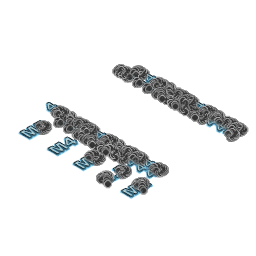
Screw-Measuring-Tool-50mm-M5_labels-only (Autodesk Fusion 360 design; units mm, degrees)
Autodesk Fusion 360 part; units mm, degrees
(part 1 of 3)
sketch "sketch 3553" plane through (0, 0, 10) normal (0, 0, 1) x (1, 0, 0)
  line L0 (16.5014, -8.6639) -> (16.5014, -9.6)
  line L1 (16.5014, -9.6) -> (15.3999, -8.6639)
  line L2 (15.3999, -8.6639) -> (16.5014, -8.6639)
  line L3 (17.91, -7.8164) -> (17.91, -8.6639)
  line L4 (17.2558, -7.8164) -> (17.91, -7.8164)
  line L5 (17.2558, -7.3771) -> (17.2558, -7.8164)
  line L6 (16.5014, -7.3771) -> (17.2558, -7.3771)
  line L7 (16.5014, -7.8164) -> (16.5014, -7.3771)
  line L8 (14.3503, -7.8164) -> (16.5014, -7.8164)
  line L9 (14.3503, -8.6639) -> (14.3503, -7.8164)
  line L10 (16.456, -10.4354) -> (14.3503, -8.6639)
  line L11 (17.2558, -10.4354) -> (16.456, -10.4354)
  line L12 (17.2558, -8.6639) -> (17.2558, -10.4354)
  line L13 (17.91, -8.6639) -> (17.2558, -8.6639)
  line L14 (16.5014, -11.9252) -> (16.5014, -12.8612)
  line L15 (16.5014, -12.8612) -> (15.3999, -11.9252)
  line L16 (15.3999, -11.9252) -> (16.5014, -11.9252)
  line L17 (17.91, -11.0777) -> (17.91, -11.9252)
  line L18 (17.2558, -11.0777) -> (17.91, -11.0777)
  line L19 (17.2558, -10.6384) -> (17.2558, -11.0777)
  line L20 (16.5014, -10.6384) -> (17.2558, -10.6384)
  line L21 (16.5014, -11.0777) -> (16.5014, -10.6384)
  line L22 (14.3503, -11.0777) -> (16.5014, -11.0777)
  line L23 (14.3503, -11.9252) -> (14.3503, -11.0777)
  line L24 (16.456, -13.6967) -> (14.3503, -11.9252)
  line L25 (17.2558, -13.6967) -> (16.456, -13.6967)
  line L26 (17.2558, -11.9252) -> (17.2558, -13.6967)
  line L27 (17.91, -11.9252) -> (17.2558, -11.9252)
  line L28 (-3.4986, -8.6639) -> (-3.4986, -9.6)
  line L29 (-3.4986, -9.6) -> (-4.6001, -8.6639)
  line L30 (-4.6001, -8.6639) -> (-3.4986, -8.6639)
  line L31 (-2.09, -7.8164) -> (-2.09, -8.6639)
  line L32 (-2.7442, -7.8164) -> (-2.09, -7.8164)
  line L33 (-2.7442, -7.3771) -> (-2.7442, -7.8164)
  line L34 (-3.4986, -7.3771) -> (-2.7442, -7.3771)
  line L35 (-3.4986, -7.8164) -> (-3.4986, -7.3771)
  line L36 (-5.6497, -7.8164) -> (-3.4986, -7.8164)
  line L37 (-5.6497, -8.6639) -> (-5.6497, -7.8164)
  line L38 (-3.544, -10.4354) -> (-5.6497, -8.6639)
  line L39 (-2.7442, -10.4354) -> (-3.544, -10.4354)
  line L40 (-2.7442, -8.6639) -> (-2.7442, -10.4354)
  line L41 (-2.09, -8.6639) -> (-2.7442, -8.6639)
  spline S0 degree 2 poles (-13.0958, -12.5579) (-13.3202, -12.2833) (-13.6497, -12.1281) knots 0 0 0 1 1 1
  spline S1 degree 2 poles (-12.7114, -13.329) (-12.8714, -12.8324) (-13.0958, -12.5579) knots 0 0 0 1 1 1
  line L42 (-11.914, -13.329) -> (-12.7114, -13.329)
  spline S2 degree 2 poles (-12.1289, -12.7692) (-12.0167, -12.9924) (-11.914, -13.329) knots 0 0 0 1 1 1
  spline S3 degree 2 poles (-12.4225, -12.3072) (-12.2411, -12.5459) (-12.1289, -12.7692) knots 0 0 0 1 1 1
  line L43 (-10.09, -12.3072) -> (-12.4225, -12.3072)
  line L44 (-10.09, -11.3236) -> (-10.09, -12.3072)
  line L45 (-13.6497, -11.3236) -> (-10.09, -11.3236)
  line L46 (-13.6497, -12.1281) -> (-13.6497, -11.3236)
  line L47 (-14.8826, -8.8955) -> (-14.8826, -7.3771)
  spline S4 degree 2 poles (-15.0951, -8.6627) (-15.0139, -8.7618) (-14.8826, -8.8955) knots 0 0 0 1 1 1
  spline S5 degree 2 poles (-15.3792, -8.27) (-15.1763, -8.5637) (-15.0951, -8.6627) knots 0 0 0 1 1 1
  spline S6 degree 2 poles (-16.0191, -7.5884) (-15.7278, -7.7758) (-15.3792, -8.27) knots 0 0 0 1 1 1
  spline S7 degree 2 poles (-16.6302, -7.401) (-16.3103, -7.401) (-16.0191, -7.5884) knots 0 0 0 1 1 1
  spline S8 degree 2 poles (-17.1734, -7.5645) (-16.9311, -7.401) (-16.6302, -7.401) knots 0 0 0 1 1 1
  spline S9 degree 2 poles (-17.5327, -8.0134) (-17.4157, -7.7281) (-17.1734, -7.5645) knots 0 0 0 1 1 1
  spline S10 degree 2 poles (-17.6497, -8.812) (-17.6497, -8.2987) (-17.5327, -8.0134) knots 0 0 0 1 1 1
  spline S11 degree 2 poles (-17.5267, -9.5819) (-17.6497, -9.3038) (-17.6497, -8.812) knots 0 0 0 1 1 1
  spline S12 degree 2 poles (-17.1734, -10.0129) (-17.4038, -9.8601) (-17.5267, -9.5819) knots 0 0 0 1 1 1
  spline S13 degree 2 poles (-16.5324, -10.2229) (-16.943, -10.1656) (-17.1734, -10.0129) knots 0 0 0 1 1 1
  line L48 (-16.4536, -9.2489) -> (-16.5324, -10.2229)
  spline S14 degree 2 poles (-16.8666, -9.0901) (-16.7496, -9.2083) (-16.4536, -9.2489) knots 0 0 0 1 1 1
  spline S15 degree 2 poles (-16.9836, -8.7857) (-16.9836, -8.9719) (-16.8666, -9.0901) knots 0 0 0 1 1 1
  spline S16 degree 2 poles (-16.8702, -8.4885) (-16.9836, -8.6066) (-16.9836, -8.7857) knots 0 0 0 1 1 1
  spline S17 degree 2 poles (-16.5968, -8.3703) (-16.7568, -8.3703) (-16.8702, -8.4885) knots 0 0 0 1 1 1
  spline S18 degree 2 poles (-16.2841, -8.4897) (-16.4488, -8.3703) (-16.5968, -8.3703) knots 0 0 0 1 1 1
  spline S19 degree 2 poles (-15.8018, -9.0364) (-16.1193, -8.609) (-16.2841, -8.4897) knots 0 0 0 1 1 1
  spline S20 degree 2 poles (-14.9029, -9.9902) (-15.2837, -9.7359) (-15.8018, -9.0364) knots 0 0 0 1 1 1
  spline S21 degree 2 poles (-14.09, -10.2946) (-14.5221, -10.2444) (-14.9029, -9.9902) knots 0 0 0 1 1 1
  line L49 (-14.09, -7.3771) -> (-14.09, -10.2946)
  line L50 (-14.8826, -7.3771) -> (-14.09, -7.3771)
  spline S22 degree 2 poles (-20.6589, -9.2154) (-20.8356, -9.2154) (-20.9466, -9.1044) knots -1 -1 -1 0 0 0
  spline S23 degree 2 poles (-20.9466, -9.1044) (-21.0576, -8.9934) (-21.0576, -8.8167) knots -1 -1 -1 0 0 0
  spline S24 degree 2 poles (-21.0576, -8.8167) (-21.0576, -8.6425) (-20.9442, -8.5302) knots -1 -1 -1 0 0 0
  spline S25 degree 2 poles (-20.9442, -8.5302) (-20.8308, -8.418) (-20.6493, -8.418) knots -1 -1 -1 0 0 0
  spline S26 degree 2 poles (-20.6493, -8.418) (-20.4751, -8.418) (-20.3652, -8.5255) knots -1 -1 -1 0 0 0
  spline S27 degree 2 poles (-20.3652, -8.5255) (-20.2554, -8.6329) (-20.2554, -8.8) knots -1 -1 -1 0 0 0
  spline S28 degree 2 poles (-20.2554, -8.8) (-20.2554, -8.9886) (-20.3664, -9.102) knots -1 -1 -1 0 0 0
  spline S29 degree 2 poles (-20.3664, -9.102) (-20.4774, -9.2154) (-20.6589, -9.2154) knots -1 -1 -1 0 0 0
  spline S30 degree 2 poles (-19.1524, -9.268) (-19.3959, -9.268) (-19.5392, -9.1331) knots -1 -1 -1 0 0 0
  spline S31 degree 2 poles (-19.5392, -9.1331) (-19.6824, -8.9982) (-19.6824, -8.8167) knots -1 -1 -1 0 0 0
  spline S32 degree 2 poles (-19.6824, -8.8167) (-19.6824, -8.6329) (-19.5344, -8.4932) knots -1 -1 -1 0 0 0
  spline S33 degree 2 poles (-19.5344, -8.4932) (-19.3864, -8.3536) (-19.1548, -8.3536) knots -1 -1 -1 0 0 0
  spline S34 degree 2 poles (-19.1548, -8.3536) (-18.9256, -8.3536) (-18.7764, -8.492) knots -1 -1 -1 0 0 0
  spline S35 degree 2 poles (-18.7764, -8.492) (-18.6272, -8.6305) (-18.6272, -8.8048) knots -1 -1 -1 0 0 0
  spline S36 degree 2 poles (-18.6272, -8.8048) (-18.6272, -8.9862) (-18.774, -9.1271) knots -1 -1 -1 0 0 0
  spline S37 degree 2 poles (-18.774, -9.1271) (-18.9208, -9.268) (-19.1524, -9.268) knots -1 -1 -1 0 0 0
  spline S38 degree 2 poles (-19.119, -10.2373) (-19.427, -10.2373) (-19.6406, -10.094) knots 0 0 0 1 1 1
  spline S39 degree 2 poles (-18.5484, -10.0845) (-18.8038, -10.2373) (-19.119, -10.2373) knots 0 0 0 1 1 1
  spline S40 degree 2 poles (-18.1616, -9.638) (-18.2929, -9.9317) (-18.5484, -10.0845) knots 0 0 0 1 1 1
  spline S41 degree 2 poles (-18.0303, -8.7881) (-18.0303, -9.3444) (-18.1616, -9.638) knots 0 0 0 1 1 1
  spline S42 degree 2 poles (-18.0888, -8.2306) (-18.0303, -8.492) (-18.0303, -8.7881) knots 0 0 0 1 1 1
  spline S43 degree 2 poles (-18.2714, -7.7937) (-18.1473, -7.9692) (-18.0888, -8.2306) knots 0 0 0 1 1 1
  spline S44 degree 2 poles (-18.6236, -7.4977) (-18.3956, -7.6182) (-18.2714, -7.7937) knots 0 0 0 1 1 1
  spline S45 degree 2 poles (-19.1142, -7.3771) (-18.8516, -7.3771) (-18.6236, -7.4977) knots 0 0 0 1 1 1
  spline S46 degree 2 poles (-19.6108, -7.5168) (-19.3864, -7.3771) (-19.1142, -7.3771) knots 0 0 0 1 1 1
  spline S47 degree 2 poles (-19.9713, -7.9405) (-19.8352, -7.6564) (-19.6108, -7.5168) knots 0 0 0 1 1 1
  spline S48 degree 2 poles (-20.2674, -7.6254) (-20.1146, -7.7257) (-19.9713, -7.9405) knots 0 0 0 1 1 1
  spline S49 degree 2 poles (-20.709, -7.4917) (-20.4727, -7.4917) (-20.2674, -7.6254) knots 0 0 0 1 1 1
  spline S50 degree 2 poles (-21.3823, -7.8271) (-21.1149, -7.4917) (-20.709, -7.4917) knots 0 0 0 1 1 1
  spline S51 degree 2 poles (-21.6497, -8.8645) (-21.6497, -8.1626) (-21.3823, -7.8271) knots 0 0 0 1 1 1
  spline S52 degree 2 poles (-21.4348, -9.7168) (-21.6497, -9.3945) (-21.6497, -8.8645) knots 0 0 0 1 1 1
  spline S53 degree 2 poles (-20.7162, -10.1298) (-21.1555, -10.1298) (-21.4348, -9.7168) knots 0 0 0 1 1 1
  spline S54 degree 2 poles (-20.2435, -9.9866) (-20.4488, -10.1298) (-20.7162, -10.1298) knots 0 0 0 1 1 1
  spline S55 degree 2 poles (-19.9713, -9.6523) (-20.0931, -9.8815) (-20.2435, -9.9866) knots 0 0 0 1 1 1
  spline S56 degree 2 poles (-19.6406, -10.094) (-19.8543, -9.9508) (-19.9713, -9.6523) knots 0 0 0 1 1 1
  line L51 (1.1174, -12.1711) -> (1.1174, -10.6527)
  spline S57 degree 2 poles (0.9049, -11.9383) (0.9861, -12.0374) (1.1174, -12.1711) knots 0 0 0 1 1 1
  spline S58 degree 2 poles (0.6208, -11.5456) (0.8237, -11.8392) (0.9049, -11.9383) knots 0 0 0 1 1 1
  spline S59 degree 2 poles (-0.0191, -10.864) (0.2722, -11.0514) (0.6208, -11.5456) knots 0 0 0 1 1 1
  spline S60 degree 2 poles (-0.6302, -10.6766) (-0.3103, -10.6766) (-0.0191, -10.864) knots 0 0 0 1 1 1
  spline S61 degree 2 poles (-1.1734, -10.8401) (-0.9311, -10.6766) (-0.6302, -10.6766) knots 0 0 0 1 1 1
  spline S62 degree 2 poles (-1.5327, -11.2889) (-1.4157, -11.0036) (-1.1734, -10.8401) knots 0 0 0 1 1 1
  spline S63 degree 2 poles (-1.6497, -12.0875) (-1.6497, -11.5742) (-1.5327, -11.2889) knots 0 0 0 1 1 1
  spline S64 degree 2 poles (-1.5267, -12.8575) (-1.6497, -12.5794) (-1.6497, -12.0875) knots 0 0 0 1 1 1
  spline S65 degree 2 poles (-1.1734, -13.2884) (-1.4038, -13.1356) (-1.5267, -12.8575) knots 0 0 0 1 1 1
  spline S66 degree 2 poles (-0.5324, -13.4985) (-0.943, -13.4412) (-1.1734, -13.2884) knots 0 0 0 1 1 1
  line L52 (-0.4536, -12.5244) -> (-0.5324, -13.4985)
  spline S67 degree 2 poles (-0.8666, -12.3657) (-0.7496, -12.4839) (-0.4536, -12.5244) knots 0 0 0 1 1 1
  spline S68 degree 2 poles (-0.9836, -12.0613) (-0.9836, -12.2475) (-0.8666, -12.3657) knots 0 0 0 1 1 1
  spline S69 degree 2 poles (-0.8702, -11.764) (-0.9836, -11.8822) (-0.9836, -12.0613) knots 0 0 0 1 1 1
  spline S70 degree 2 poles (-0.5968, -11.6459) (-0.7568, -11.6459) (-0.8702, -11.764) knots 0 0 0 1 1 1
  spline S71 degree 2 poles (-0.2841, -11.7652) (-0.4488, -11.6459) (-0.5968, -11.6459) knots 0 0 0 1 1 1
  spline S72 degree 2 poles (0.1982, -12.312) (-0.1193, -11.8846) (-0.2841, -11.7652) knots 0 0 0 1 1 1
  spline S73 degree 2 poles (1.0971, -13.2657) (0.7163, -13.0115) (0.1982, -12.312) knots 0 0 0 1 1 1
  spline S74 degree 2 poles (1.91, -13.5701) (1.4779, -13.52) (1.0971, -13.2657) knots 0 0 0 1 1 1
  line L53 (1.91, -10.6527) -> (1.91, -13.5701)
  line L54 (1.1174, -10.6527) -> (1.91, -10.6527)
  spline S75 degree 2 poles (6.9543, -12.1592) (6.9543, -12.3311) (7.0582, -12.4385) knots 0 0 0 1 1 1
  spline S76 degree 2 poles (7.0498, -11.8965) (6.9543, -11.992) (6.9543, -12.1592) knots 0 0 0 1 1 1
  spline S77 degree 2 poles (7.3053, -11.801) (7.1453, -11.801) (7.0498, -11.8965) knots 0 0 0 1 1 1
  spline S78 degree 2 poles (7.5942, -11.9288) (7.4724, -11.801) (7.3053, -11.801) knots 0 0 0 1 1 1
  spline S79 degree 2 poles (7.7159, -12.2475) (7.7159, -12.0565) (7.5942, -11.9288) knots 0 0 0 1 1 1
  spline S80 degree 2 poles (7.704, -12.374) (7.7159, -12.2929) (7.7159, -12.2475) knots 0 0 0 1 1 1
  line L55 (8.3987, -12.4242) -> (7.704, -12.374)
  spline S81 degree 2 poles (8.3414, -12.109) (8.3414, -12.2236) (8.3987, -12.4242) knots 0 0 0 1 1 1
  spline S82 degree 2 poles (8.4751, -11.7688) (8.3414, -11.8942) (8.3414, -12.109) knots 0 0 0 1 1 1
  spline S83 degree 2 poles (8.8524, -11.6435) (8.6088, -11.6435) (8.4751, -11.7688) knots 0 0 0 1 1 1
  spline S84 degree 2 poles (9.2344, -11.7736) (9.0911, -11.6435) (8.8524, -11.6435) knots 0 0 0 1 1 1
  spline S85 degree 2 poles (9.3776, -12.0995) (9.3776, -11.9037) (9.2344, -11.7736) knots 0 0 0 1 1 1
  spline S86 degree 2 poles (9.2642, -12.4063) (9.3776, -12.2857) (9.3776, -12.0995) knots 0 0 0 1 1 1
  spline S87 degree 2 poles (8.8571, -12.5841) (9.1508, -12.5268) (9.2642, -12.4063) knots 0 0 0 1 1 1
  line L56 (8.9861, -13.5558) -> (8.8571, -12.5841)
  spline S88 degree 2 poles (9.5292, -13.2825) (9.3131, -13.4603) (8.9861, -13.5558) knots 0 0 0 1 1 1
  spline S89 degree 2 poles (9.8575, -12.8288) (9.7453, -13.1046) (9.5292, -13.2825) knots 0 0 0 1 1 1
  spline S90 degree 2 poles (9.9697, -12.0756) (9.9697, -12.5531) (9.8575, -12.8288) knots 0 0 0 1 1 1
  spline S91 degree 2 poles (9.8181, -11.2854) (9.9697, -11.5862) (9.9697, -12.0756) knots 0 0 0 1 1 1
  spline S92 degree 2 poles (9.386, -10.8246) (9.6665, -10.9845) (9.8181, -11.2854) knots 0 0 0 1 1 1
  spline S93 degree 2 poles (8.7998, -10.6646) (9.1054, -10.6646) (9.386, -10.8246) knots 0 0 0 1 1 1
  spline S94 degree 2 poles (8.3808, -10.7613) (8.5563, -10.6646) (8.7998, -10.6646) knots 0 0 0 1 1 1
  spline S95 degree 2 poles (8.0979, -11.0323) (8.2054, -10.858) (8.3808, -10.7613) knots 0 0 0 1 1 1
  spline S96 degree 2 poles (7.9809, -11.3427) (8.0311, -11.1397) (8.0979, -11.0323) knots 0 0 0 1 1 1
  spline S97 degree 2 poles (7.6586, -10.9678) (7.8425, -11.092) (7.9809, -11.3427) knots 0 0 0 1 1 1
  spline S98 degree 2 poles (7.248, -10.8437) (7.4748, -10.8437) (7.6586, -10.9678) knots 0 0 0 1 1 1
  spline S99 degree 2 poles (6.6058, -11.1493) (6.8612, -10.8437) (7.248, -10.8437) knots 0 0 0 1 1 1
  spline S100 degree 2 poles (6.3503, -12.1401) (6.3503, -11.4549) (6.6058, -11.1493) knots 0 0 0 1 1 1
  spline S101 degree 2 poles (6.5843, -13.0628) (6.3503, -12.7369) (6.3503, -12.1401) knots 0 0 0 1 1 1
  spline S102 degree 2 poles (7.2575, -13.5033) (6.8183, -13.3887) (6.5843, -13.0628) knots 0 0 0 1 1 1
  line L57 (7.4223, -12.5841) -> (7.2575, -13.5033)
  spline S103 degree 2 poles (7.0582, -12.4385) (7.162, -12.5459) (7.4223, -12.5841) knots 0 0 0 1 1 1
  spline S104 degree 2 poles (20.8476, -9.268) (20.6041, -9.268) (20.4608, -9.1331) knots -1 -1 -1 0 0 0
  spline S105 degree 2 poles (20.4608, -9.1331) (20.3176, -8.9982) (20.3176, -8.8167) knots -1 -1 -1 0 0 0
  spline S106 degree 2 poles (20.3176, -8.8167) (20.3176, -8.6329) (20.4656, -8.4932) knots -1 -1 -1 0 0 0
  spline S107 degree 2 poles (20.4656, -8.4932) (20.6136, -8.3536) (20.8452, -8.3536) knots -1 -1 -1 0 0 0
  spline S108 degree 2 poles (20.8452, -8.3536) (21.0744, -8.3536) (21.2236, -8.492) knots -1 -1 -1 0 0 0
  spline S109 degree 2 poles (21.2236, -8.492) (21.3728, -8.6305) (21.3728, -8.8048) knots -1 -1 -1 0 0 0
  spline S110 degree 2 poles (21.3728, -8.8048) (21.3728, -8.9862) (21.226, -9.1271) knots -1 -1 -1 0 0 0
  spline S111 degree 2 poles (21.226, -9.1271) (21.0792, -9.268) (20.8476, -9.268) knots -1 -1 -1 0 0 0
  spline S112 degree 2 poles (19.3411, -9.2154) (19.1644, -9.2154) (19.0534, -9.1044) knots -1 -1 -1 0 0 0
  spline S113 degree 2 poles (19.0534, -9.1044) (18.9424, -8.9934) (18.9424, -8.8167) knots -1 -1 -1 0 0 0
  spline S114 degree 2 poles (18.9424, -8.8167) (18.9424, -8.6425) (19.0558, -8.5302) knots -1 -1 -1 0 0 0
  spline S115 degree 2 poles (19.0558, -8.5302) (19.1692, -8.418) (19.3507, -8.418) knots -1 -1 -1 0 0 0
  spline S116 degree 2 poles (19.3507, -8.418) (19.5249, -8.418) (19.6348, -8.5255) knots -1 -1 -1 0 0 0
  spline S117 degree 2 poles (19.6348, -8.5255) (19.7446, -8.6329) (19.7446, -8.8) knots -1 -1 -1 0 0 0
  spline S118 degree 2 poles (19.7446, -8.8) (19.7446, -8.9886) (19.6336, -9.102) knots -1 -1 -1 0 0 0
  spline S119 degree 2 poles (19.6336, -9.102) (19.5226, -9.2154) (19.3411, -9.2154) knots -1 -1 -1 0 0 0
  spline S120 degree 2 poles (20.881, -10.2373) (20.573, -10.2373) (20.3594, -10.094) knots 0 0 0 1 1 1
  spline S121 degree 2 poles (21.4516, -10.0845) (21.1962, -10.2373) (20.881, -10.2373) knots 0 0 0 1 1 1
  spline S122 degree 2 poles (21.8384, -9.638) (21.7071, -9.9317) (21.4516, -10.0845) knots 0 0 0 1 1 1
  spline S123 degree 2 poles (21.9697, -8.7881) (21.9697, -9.3444) (21.8384, -9.638) knots 0 0 0 1 1 1
  spline S124 degree 2 poles (21.9112, -8.2306) (21.9697, -8.492) (21.9697, -8.7881) knots 0 0 0 1 1 1
  spline S125 degree 2 poles (21.7286, -7.7937) (21.8527, -7.9692) (21.9112, -8.2306) knots 0 0 0 1 1 1
  spline S126 degree 2 poles (21.3764, -7.4977) (21.6044, -7.6182) (21.7286, -7.7937) knots 0 0 0 1 1 1
  spline S127 degree 2 poles (20.8858, -7.3771) (21.1484, -7.3771) (21.3764, -7.4977) knots 0 0 0 1 1 1
  spline S128 degree 2 poles (20.3892, -7.5168) (20.6136, -7.3771) (20.8858, -7.3771) knots 0 0 0 1 1 1
  spline S129 degree 2 poles (20.0287, -7.9405) (20.1648, -7.6564) (20.3892, -7.5168) knots 0 0 0 1 1 1
  spline S130 degree 2 poles (19.7326, -7.6254) (19.8854, -7.7257) (20.0287, -7.9405) knots 0 0 0 1 1 1
  spline S131 degree 2 poles (19.291, -7.4917) (19.5273, -7.4917) (19.7326, -7.6254) knots 0 0 0 1 1 1
  spline S132 degree 2 poles (18.6177, -7.8271) (18.8851, -7.4917) (19.291, -7.4917) knots 0 0 0 1 1 1
  spline S133 degree 2 poles (18.3503, -8.8645) (18.3503, -8.1626) (18.6177, -7.8271) knots 0 0 0 1 1 1
  spline S134 degree 2 poles (18.5652, -9.7168) (18.3503, -9.3945) (18.3503, -8.8645) knots 0 0 0 1 1 1
  spline S135 degree 2 poles (19.2838, -10.1298) (18.8445, -10.1298) (18.5652, -9.7168) knots 0 0 0 1 1 1
  spline S136 degree 2 poles (19.7565, -9.9866) (19.5512, -10.1298) (19.2838, -10.1298) knots 0 0 0 1 1 1
  spline S137 degree 2 poles (20.0287, -9.6523) (19.9069, -9.8815) (19.7565, -9.9866) knots 0 0 0 1 1 1
  spline S138 degree 2 poles (20.3594, -10.094) (20.1457, -9.9508) (20.0287, -9.6523) knots 0 0 0 1 1 1
  line L58 (-6.8826, -12.1711) -> (-6.8826, -10.6527)
  spline S139 degree 2 poles (-7.0951, -11.9383) (-7.0139, -12.0374) (-6.8826, -12.1711) knots 0 0 0 1 1 1
  spline S140 degree 2 poles (-7.3792, -11.5456) (-7.1763, -11.8392) (-7.0951, -11.9383) knots 0 0 0 1 1 1
  spline S141 degree 2 poles (-8.0191, -10.864) (-7.7278, -11.0514) (-7.3792, -11.5456) knots 0 0 0 1 1 1
  spline S142 degree 2 poles (-8.6302, -10.6766) (-8.3103, -10.6766) (-8.0191, -10.864) knots 0 0 0 1 1 1
  spline S143 degree 2 poles (-9.1734, -10.8401) (-8.9311, -10.6766) (-8.6302, -10.6766) knots 0 0 0 1 1 1
  spline S144 degree 2 poles (-9.5327, -11.2889) (-9.4157, -11.0036) (-9.1734, -10.8401) knots 0 0 0 1 1 1
  spline S145 degree 2 poles (-9.6497, -12.0875) (-9.6497, -11.5742) (-9.5327, -11.2889) knots 0 0 0 1 1 1
  spline S146 degree 2 poles (-9.5267, -12.8575) (-9.6497, -12.5794) (-9.6497, -12.0875) knots 0 0 0 1 1 1
  spline S147 degree 2 poles (-9.1734, -13.2884) (-9.4038, -13.1356) (-9.5267, -12.8575) knots 0 0 0 1 1 1
  spline S148 degree 2 poles (-8.5324, -13.4985) (-8.943, -13.4412) (-9.1734, -13.2884) knots 0 0 0 1 1 1
  line L59 (-8.4536, -12.5244) -> (-8.5324, -13.4985)
  spline S149 degree 2 poles (-8.8666, -12.3657) (-8.7496, -12.4839) (-8.4536, -12.5244) knots 0 0 0 1 1 1
  spline S150 degree 2 poles (-8.9836, -12.0613) (-8.9836, -12.2475) (-8.8666, -12.3657) knots 0 0 0 1 1 1
  spline S151 degree 2 poles (-8.8702, -11.764) (-8.9836, -11.8822) (-8.9836, -12.0613) knots 0 0 0 1 1 1
  spline S152 degree 2 poles (-8.5968, -11.6459) (-8.7568, -11.6459) (-8.8702, -11.764) knots 0 0 0 1 1 1
  spline S153 degree 2 poles (-8.2841, -11.7652) (-8.4488, -11.6459) (-8.5968, -11.6459) knots 0 0 0 1 1 1
  spline S154 degree 2 poles (-7.8018, -12.312) (-8.1193, -11.8846) (-8.2841, -11.7652) knots 0 0 0 1 1 1
  spline S155 degree 2 poles (-6.9029, -13.2657) (-7.2837, -13.0115) (-7.8018, -12.312) knots 0 0 0 1 1 1
  spline S156 degree 2 poles (-6.09, -13.5701) (-6.5221, -13.52) (-6.9029, -13.2657) knots 0 0 0 1 1 1
  line L60 (-6.09, -10.6527) -> (-6.09, -13.5701)
  line L61 (-6.8826, -10.6527) -> (-6.09, -10.6527)
  line L62 (5.1174, -8.8955) -> (5.1174, -7.3771)
  spline S157 degree 2 poles (4.9049, -8.6627) (4.9861, -8.7618) (5.1174, -8.8955) knots 0 0 0 1 1 1
  spline S158 degree 2 poles (4.6208, -8.27) (4.8237, -8.5637) (4.9049, -8.6627) knots 0 0 0 1 1 1
  spline S159 degree 2 poles (3.9809, -7.5884) (4.2722, -7.7758) (4.6208, -8.27) knots 0 0 0 1 1 1
  spline S160 degree 2 poles (3.3698, -7.401) (3.6897, -7.401) (3.9809, -7.5884) knots 0 0 0 1 1 1
  spline S161 degree 2 poles (2.8266, -7.5645) (3.0689, -7.401) (3.3698, -7.401) knots 0 0 0 1 1 1
  spline S162 degree 2 poles (2.4673, -8.0134) (2.5843, -7.7281) (2.8266, -7.5645) knots 0 0 0 1 1 1
  spline S163 degree 2 poles (2.3503, -8.812) (2.3503, -8.2987) (2.4673, -8.0134) knots 0 0 0 1 1 1
  spline S164 degree 2 poles (2.4733, -9.5819) (2.3503, -9.3038) (2.3503, -8.812) knots 0 0 0 1 1 1
  spline S165 degree 2 poles (2.8266, -10.0129) (2.5962, -9.8601) (2.4733, -9.5819) knots 0 0 0 1 1 1
  spline S166 degree 2 poles (3.4676, -10.2229) (3.057, -10.1656) (2.8266, -10.0129) knots 0 0 0 1 1 1
  line L63 (3.5464, -9.2489) -> (3.4676, -10.2229)
  spline S167 degree 2 poles (3.1334, -9.0901) (3.2504, -9.2083) (3.5464, -9.2489) knots 0 0 0 1 1 1
  spline S168 degree 2 poles (3.0164, -8.7857) (3.0164, -8.9719) (3.1334, -9.0901) knots 0 0 0 1 1 1
  spline S169 degree 2 poles (3.1298, -8.4885) (3.0164, -8.6066) (3.0164, -8.7857) knots 0 0 0 1 1 1
  spline S170 degree 2 poles (3.4032, -8.3703) (3.2432, -8.3703) (3.1298, -8.4885) knots 0 0 0 1 1 1
  spline S171 degree 2 poles (3.7159, -8.4897) (3.5512, -8.3703) (3.4032, -8.3703) knots 0 0 0 1 1 1
  spline S172 degree 2 poles (4.1982, -9.0364) (3.8807, -8.609) (3.7159, -8.4897) knots 0 0 0 1 1 1
  spline S173 degree 2 poles (5.0971, -9.9902) (4.7163, -9.7359) (4.1982, -9.0364) knots 0 0 0 1 1 1
  spline S174 degree 2 poles (5.91, -10.2946) (5.4779, -10.2444) (5.0971, -9.9902) knots 0 0 0 1 1 1
  line L64 (5.91, -7.3771) -> (5.91, -10.2946)
  line L65 (5.1174, -7.3771) -> (5.91, -7.3771)
  spline S175 degree 2 poles (-15.0958, 17.7183) (-15.3202, 17.9928) (-15.6497, 18.148) knots 0 0 0 1 1 1
  spline S176 degree 2 poles (-14.7114, 16.9471) (-14.8714, 17.4437) (-15.0958, 17.7183) knots 0 0 0 1 1 1
  line L66 (-13.914, 16.9471) -> (-14.7114, 16.9471)
  spline S177 degree 2 poles (-14.1289, 17.507) (-14.0167, 17.2837) (-13.914, 16.9471) knots 0 0 0 1 1 1
  spline S178 degree 2 poles (-14.4225, 17.9689) (-14.2411, 17.7302) (-14.1289, 17.507) knots 0 0 0 1 1 1
  line L67 (-12.09, 17.9689) -> (-14.4225, 17.9689)
  line L68 (-12.09, 18.9526) -> (-12.09, 17.9689)
  line L69 (-15.6497, 18.9526) -> (-12.09, 18.9526)
  line L70 (-15.6497, 18.148) -> (-15.6497, 18.9526)
  line L71 (-13.4986, 21.6814) -> (-13.4986, 20.7454)
  line L72 (-13.4986, 20.7454) -> (-14.6001, 21.6814)
  line L73 (-14.6001, 21.6814) -> (-13.4986, 21.6814)
  line L74 (-12.09, 22.529) -> (-12.09, 21.6814)
  line L75 (-12.7442, 22.529) -> (-12.09, 22.529)
  line L76 (-12.7442, 22.9683) -> (-12.7442, 22.529)
  line L77 (-13.4986, 22.9683) -> (-12.7442, 22.9683)
  line L78 (-13.4986, 22.529) -> (-13.4986, 22.9683)
  line L79 (-15.6497, 22.529) -> (-13.4986, 22.529)
  line L80 (-15.6497, 21.6814) -> (-15.6497, 22.529)
  line L81 (-13.544, 19.9099) -> (-15.6497, 21.6814)
  line L82 (-12.7442, 19.9099) -> (-13.544, 19.9099)
  line L83 (-12.7442, 21.6814) -> (-12.7442, 19.9099)
  line L84 (-12.09, 21.6814) -> (-12.7442, 21.6814)
  spline S179 degree 2 poles (-19.0958, 17.7183) (-19.3202, 17.9928) (-19.6497, 18.148) knots 0 0 0 1 1 1
  spline S180 degree 2 poles (-18.7114, 16.9471) (-18.8714, 17.4437) (-19.0958, 17.7183) knots 0 0 0 1 1 1
  line L85 (-17.914, 16.9471) -> (-18.7114, 16.9471)
  spline S181 degree 2 poles (-18.1289, 17.507) (-18.0167, 17.2837) (-17.914, 16.9471) knots 0 0 0 1 1 1
  spline S182 degree 2 poles (-18.4225, 17.9689) (-18.2411, 17.7302) (-18.1289, 17.507) knots 0 0 0 1 1 1
  line L86 (-16.09, 17.9689) -> (-18.4225, 17.9689)
  line L87 (-16.09, 18.9526) -> (-16.09, 17.9689)
  line L88 (-19.6497, 18.9526) -> (-16.09, 18.9526)
  line L89 (-19.6497, 18.148) -> (-19.6497, 18.9526)
  spline S183 degree 2 poles (-21.2431, 17.9665) (-21.5225, 17.9665) (-21.6729, 18.1038) knots -1 -1 -1 0 0 0
  spline S184 degree 2 poles (-21.6729, 18.1038) (-21.8233, 18.2411) (-21.8233, 18.444) knots -1 -1 -1 0 0 0
  spline S185 degree 2 poles (-21.8233, 18.444) (-21.8233, 18.6422) (-21.6681, 18.7759) knots -1 -1 -1 0 0 0
  spline S186 degree 2 poles (-21.6681, 18.7759) (-21.5129, 18.9096) (-21.2169, 18.9096) knots -1 -1 -1 0 0 0
  spline S187 degree 2 poles (-21.2169, 18.9096) (-20.928, 18.9096) (-20.7824, 18.7807) knots -1 -1 -1 0 0 0
  spline S188 degree 2 poles (-20.7824, 18.7807) (-20.6367, 18.6517) (-20.6367, 18.4607) knots -1 -1 -1 0 0 0
  spline S189 degree 2 poles (-20.6367, 18.4607) (-20.6367, 18.253) (-20.7979, 18.1098) knots -1 -1 -1 0 0 0
  spline S190 degree 2 poles (-20.7979, 18.1098) (-20.959, 17.9665) (-21.2431, 17.9665) knots -1 -1 -1 0 0 0
  spline S191 degree 2 poles (-23.553, 19.1113) (-23.4563, 19.3537) (-23.2701, 19.5136) knots 0 0 0 1 1 1
  spline S192 degree 2 poles (-23.6497, 18.4512) (-23.6497, 18.869) (-23.553, 19.1113) knots 0 0 0 1 1 1
  spline S193 degree 2 poles (-23.2092, 17.3458) (-23.6497, 17.7445) (-23.6497, 18.4512) knots 0 0 0 1 1 1
  spline S194 degree 2 poles (-21.8209, 16.9471) (-22.7687, 16.9471) (-23.2092, 17.3458) knots 0 0 0 1 1 1
  spline S195 degree 2 poles (-20.7812, 17.1369) (-21.1739, 16.9471) (-21.8209, 16.9471) knots 0 0 0 1 1 1
  spline S196 degree 2 poles (-20.2094, 17.6442) (-20.3884, 17.3267) (-20.7812, 17.1369) knots 0 0 0 1 1 1
  spline S197 degree 2 poles (-20.0303, 18.487) (-20.0303, 17.9618) (-20.2094, 17.6442) knots 0 0 0 1 1 1
  spline S198 degree 2 poles (-20.1771, 19.214) (-20.0303, 18.9239) (-20.0303, 18.487) knots 0 0 0 1 1 1
  spline S199 degree 2 poles (-20.6105, 19.6676) (-20.324, 19.5041) (-20.1771, 19.214) knots 0 0 0 1 1 1
  spline S200 degree 2 poles (-21.2431, 19.8311) (-20.897, 19.8311) (-20.6105, 19.6676) knots 0 0 0 1 1 1
  spline S201 degree 2 poles (-22.0907, 19.5076) (-21.7564, 19.8311) (-21.2431, 19.8311) knots 0 0 0 1 1 1
  spline S202 degree 2 poles (-22.4249, 18.7162) (-22.4249, 19.1841) (-22.0907, 19.5076) knots 0 0 0 1 1 1
  spline S203 degree 2 poles (-22.3402, 18.2912) (-22.4249, 18.4751) (-22.4249, 18.7162) knots 0 0 0 1 1 1
  spline S204 degree 2 poles (-22.0787, 17.9331) (-22.2554, 18.1074) (-22.3402, 18.2912) knots 0 0 0 1 1 1
  spline S205 degree 2 poles (-22.8141, 18.074) (-22.6422, 17.9785) (-22.0787, 17.9331) knots 0 0 0 1 1 1
  spline S206 degree 2 poles (-23.0528, 18.4416) (-23.0528, 18.2053) (-22.8141, 18.074) knots 0 0 0 1 1 1
  spline S207 degree 2 poles (-22.9693, 18.6625) (-23.0528, 18.573) (-23.0528, 18.4416) knots 0 0 0 1 1 1
  spline S208 degree 2 poles (-22.6828, 18.7902) (-22.8857, 18.752) (-22.9693, 18.6625) knots 0 0 0 1 1 1
  line L90 (-22.8021, 19.7571) -> (-22.6828, 18.7902)
  spline S209 degree 2 poles (-23.2701, 19.5136) (-23.0839, 19.6736) (-22.8021, 19.7571) knots 0 0 0 1 1 1
  spline S210 degree 2 poles (18.7569, 21.3329) (18.4775, 21.3329) (18.3271, 21.4701) knots -1 -1 -1 0 0 0
  spline S211 degree 2 poles (18.3271, 21.4701) (18.1767, 21.6074) (18.1767, 21.8103) knots -1 -1 -1 0 0 0
  spline S212 degree 2 poles (18.1767, 21.8103) (18.1767, 22.0085) (18.3319, 22.1422) knots -1 -1 -1 0 0 0
  spline S213 degree 2 poles (18.3319, 22.1422) (18.4871, 22.2759) (18.7831, 22.2759) knots -1 -1 -1 0 0 0
  spline S214 degree 2 poles (18.7831, 22.2759) (19.072, 22.2759) (19.2176, 22.147) knots -1 -1 -1 0 0 0
  spline S215 degree 2 poles (19.2176, 22.147) (19.3633, 22.018) (19.3633, 21.8271) knots -1 -1 -1 0 0 0
  spline S216 degree 2 poles (19.3633, 21.8271) (19.3633, 21.6193) (19.2021, 21.4761) knots -1 -1 -1 0 0 0
  spline S217 degree 2 poles (19.2021, 21.4761) (19.041, 21.3329) (18.7569, 21.3329) knots -1 -1 -1 0 0 0
  spline S218 degree 2 poles (16.447, 22.4776) (16.5437, 22.72) (16.7299, 22.8799) knots 0 0 0 1 1 1
  spline S219 degree 2 poles (16.3503, 21.8175) (16.3503, 22.2353) (16.447, 22.4776) knots 0 0 0 1 1 1
  spline S220 degree 2 poles (16.7908, 20.7121) (16.3503, 21.1108) (16.3503, 21.8175) knots 0 0 0 1 1 1
  spline S221 degree 2 poles (18.1791, 20.3134) (17.2313, 20.3134) (16.7908, 20.7121) knots 0 0 0 1 1 1
  spline S222 degree 2 poles (19.2188, 20.5032) (18.8261, 20.3134) (18.1791, 20.3134) knots 0 0 0 1 1 1
  spline S223 degree 2 poles (19.7906, 21.0105) (19.6116, 20.693) (19.2188, 20.5032) knots 0 0 0 1 1 1
  spline S224 degree 2 poles (19.9697, 21.8533) (19.9697, 21.3281) (19.7906, 21.0105) knots 0 0 0 1 1 1
  spline S225 degree 2 poles (19.8229, 22.5803) (19.9697, 22.2902) (19.9697, 21.8533) knots 0 0 0 1 1 1
  spline S226 degree 2 poles (19.3895, 23.0339) (19.676, 22.8704) (19.8229, 22.5803) knots 0 0 0 1 1 1
  spline S227 degree 2 poles (18.7569, 23.1974) (19.103, 23.1974) (19.3895, 23.0339) knots 0 0 0 1 1 1
  spline S228 degree 2 poles (17.9093, 22.8739) (18.2436, 23.1974) (18.7569, 23.1974) knots 0 0 0 1 1 1
  spline S229 degree 2 poles (17.5751, 22.0825) (17.5751, 22.5504) (17.9093, 22.8739) knots 0 0 0 1 1 1
  spline S230 degree 2 poles (17.6598, 21.6575) (17.5751, 21.8414) (17.5751, 22.0825) knots 0 0 0 1 1 1
  spline S231 degree 2 poles (17.9213, 21.2994) (17.7446, 21.4737) (17.6598, 21.6575) knots 0 0 0 1 1 1
  spline S232 degree 2 poles (17.1859, 21.4403) (17.3578, 21.3448) (17.9213, 21.2994) knots 0 0 0 1 1 1
  spline S233 degree 2 poles (16.9472, 21.808) (16.9472, 21.5716) (17.1859, 21.4403) knots 0 0 0 1 1 1
  spline S234 degree 2 poles (17.0307, 22.0288) (16.9472, 21.9393) (16.9472, 21.808) knots 0 0 0 1 1 1
  spline S235 degree 2 poles (17.3172, 22.1565) (17.1143, 22.1183) (17.0307, 22.0288) knots 0 0 0 1 1 1
  line L91 (17.1979, 23.1234) -> (17.3172, 22.1565)
  spline S236 degree 2 poles (16.7299, 22.8799) (16.9161, 23.0399) (17.1979, 23.1234) knots 0 0 0 1 1 1
  spline S237 degree 2 poles (22.1481, 21.2135) (21.4867, 21.2135) (21.242, 21.3209) knots -1 -1 -1 0 0 0
  spline S238 degree 2 poles (21.242, 21.3209) (20.9973, 21.4283) (20.9973, 21.6695) knots -1 -1 -1 0 0 0
  spline S239 degree 2 poles (20.9973, 21.6695) (20.9973, 21.9058) (21.2373, 22.024) knots -1 -1 -1 0 0 0
  spline S240 degree 2 poles (21.2373, 22.024) (21.4772, 22.1422) (22.1743, 22.1422) knots -1 -1 -1 0 0 0
  spline S241 degree 2 poles (22.1743, 22.1422) (22.6494, 22.1422) (22.8738, 22.0909) knots -1 -1 -1 0 0 0
  spline S242 degree 2 poles (22.8738, 22.0909) (23.0983, 22.0395) (23.2021, 21.9309) knots -1 -1 -1 0 0 0
  spline S243 degree 2 poles (23.2021, 21.9309) (23.306, 21.8223) (23.306, 21.6743) knots -1 -1 -1 0 0 0
  spline S244 degree 2 poles (23.306, 21.6743) (23.306, 21.4498) (23.0613, 21.3317) knots -1 -1 -1 0 0 0
  spline S245 degree 2 poles (23.0613, 21.3317) (22.8165, 21.2135) (22.1481, 21.2135) knots -1 -1 -1 0 0 0
  spline S246 degree 2 poles (23.4158, 20.5163) (23.2224, 20.3898) (22.887, 20.3194) knots 0 0 0 1 1 1
  spline S247 degree 2 poles (23.8288, 20.9628) (23.688, 20.6906) (23.4158, 20.5163) knots 0 0 0 1 1 1
  spline S248 degree 2 poles (23.9697, 21.6766) (23.9697, 21.235) (23.8288, 20.9628) knots 0 0 0 1 1 1
  spline S249 degree 2 poles (23.528, 22.7868) (23.9697, 22.4645) (23.9697, 21.6766) knots 0 0 0 1 1 1
  spline S250 degree 2 poles (22.1337, 23.1091) (23.0863, 23.1091) (23.528, 22.7868) knots 0 0 0 1 1 1
  spline S251 degree 2 poles (21.3172, 23.0112) (21.7088, 23.1091) (22.1337, 23.1091) knots 0 0 0 1 1 1
  spline S252 degree 2 poles (20.9579, 22.8787) (21.1119, 22.9611) (21.3172, 23.0112) knots 0 0 0 1 1 1
  spline S253 degree 2 poles (20.6643, 22.6531) (20.8039, 22.7964) (20.9579, 22.8787) knots 0 0 0 1 1 1
  spline S254 degree 2 poles (20.4375, 22.2831) (20.5246, 22.5099) (20.6643, 22.6531) knots 0 0 0 1 1 1
  spline S255 degree 2 poles (20.3503, 21.7029) (20.3503, 22.0562) (20.4375, 22.2831) knots 0 0 0 1 1 1
  spline S256 degree 2 poles (20.749, 20.6083) (20.3503, 20.9676) (20.3503, 21.7029) knots 0 0 0 1 1 1
  spline S257 degree 2 poles (22.1457, 20.2489) (21.1477, 20.2489) (20.749, 20.6083) knots 0 0 0 1 1 1
  spline S258 degree 2 poles (22.887, 20.3194) (22.5515, 20.2489) (22.1457, 20.2489) knots 0 0 0 1 1 1
  line L92 (-0.8826, 18.3462) -> (-0.8826, 19.8646)
  spline S259 degree 2 poles (-1.0951, 18.5789) (-1.0139, 18.4798) (-0.8826, 18.3462) knots 0 0 0 1 1 1
  spline S260 degree 2 poles (-1.3792, 18.9717) (-1.1763, 18.678) (-1.0951, 18.5789) knots 0 0 0 1 1 1
  spline S261 degree 2 poles (-2.0191, 19.6533) (-1.7278, 19.4659) (-1.3792, 18.9717) knots 0 0 0 1 1 1
  spline S262 degree 2 poles (-2.6302, 19.8407) (-2.3103, 19.8407) (-2.0191, 19.6533) knots 0 0 0 1 1 1
  spline S263 degree 2 poles (-3.1734, 19.6772) (-2.9311, 19.8407) (-2.6302, 19.8407) knots 0 0 0 1 1 1
  spline S264 degree 2 poles (-3.5327, 19.2283) (-3.4157, 19.5136) (-3.1734, 19.6772) knots 0 0 0 1 1 1
  spline S265 degree 2 poles (-3.6497, 18.4297) (-3.6497, 18.943) (-3.5327, 19.2283) knots 0 0 0 1 1 1
  spline S266 degree 2 poles (-3.5267, 17.6598) (-3.6497, 17.9379) (-3.6497, 18.4297) knots 0 0 0 1 1 1
  spline S267 degree 2 poles (-3.1734, 17.2288) (-3.4038, 17.3816) (-3.5267, 17.6598) knots 0 0 0 1 1 1
  spline S268 degree 2 poles (-2.5324, 17.0187) (-2.943, 17.076) (-3.1734, 17.2288) knots 0 0 0 1 1 1
  line L93 (-2.4536, 17.9928) -> (-2.5324, 17.0187)
  spline S269 degree 2 poles (-2.8666, 18.1516) (-2.7496, 18.0334) (-2.4536, 17.9928) knots 0 0 0 1 1 1
  spline S270 degree 2 poles (-2.9836, 18.456) (-2.9836, 18.2698) (-2.8666, 18.1516) knots 0 0 0 1 1 1
  spline S271 degree 2 poles (-2.8702, 18.7532) (-2.9836, 18.635) (-2.9836, 18.456) knots 0 0 0 1 1 1
  spline S272 degree 2 poles (-2.5968, 18.8714) (-2.7568, 18.8714) (-2.8702, 18.7532) knots 0 0 0 1 1 1
  spline S273 degree 2 poles (-2.2841, 18.752) (-2.4488, 18.8714) (-2.5968, 18.8714) knots 0 0 0 1 1 1
  spline S274 degree 2 poles (-1.8018, 18.2053) (-2.1193, 18.6326) (-2.2841, 18.752) knots 0 0 0 1 1 1
  spline S275 degree 2 poles (-0.9029, 17.2515) (-1.2837, 17.5058) (-1.8018, 18.2053) knots 0 0 0 1 1 1
  spline S276 degree 2 poles (-0.09, 16.9471) (-0.5221, 16.9972) (-0.9029, 17.2515) knots 0 0 0 1 1 1
  line L94 (-0.09, 19.8646) -> (-0.09, 16.9471)
  line L95 (-0.8826, 19.8646) -> (-0.09, 19.8646)
  spline S277 degree 2 poles (4.9543, 18.3438) (4.9543, 18.1719) (5.0582, 18.0644) knots 0 0 0 1 1 1
  spline S278 degree 2 poles (5.0498, 18.6064) (4.9543, 18.5109) (4.9543, 18.3438) knots 0 0 0 1 1 1
  spline S279 degree 2 poles (5.3053, 18.7019) (5.1453, 18.7019) (5.0498, 18.6064) knots 0 0 0 1 1 1
  spline S280 degree 2 poles (5.5942, 18.5742) (5.4724, 18.7019) (5.3053, 18.7019) knots 0 0 0 1 1 1
  spline S281 degree 2 poles (5.7159, 18.2554) (5.7159, 18.4464) (5.5942, 18.5742) knots 0 0 0 1 1 1
  spline S282 degree 2 poles (5.704, 18.1289) (5.7159, 18.2101) (5.7159, 18.2554) knots 0 0 0 1 1 1
  line L96 (6.3987, 18.0788) -> (5.704, 18.1289)
  spline S283 degree 2 poles (6.3414, 18.3939) (6.3414, 18.2793) (6.3987, 18.0788) knots 0 0 0 1 1 1
  spline S284 degree 2 poles (6.4751, 18.7341) (6.3414, 18.6088) (6.3414, 18.3939) knots 0 0 0 1 1 1
  spline S285 degree 2 poles (6.8524, 18.8595) (6.6088, 18.8595) (6.4751, 18.7341) knots 0 0 0 1 1 1
  spline S286 degree 2 poles (7.2344, 18.7293) (7.0911, 18.8595) (6.8524, 18.8595) knots 0 0 0 1 1 1
  spline S287 degree 2 poles (7.3776, 18.4035) (7.3776, 18.5992) (7.2344, 18.7293) knots 0 0 0 1 1 1
  spline S288 degree 2 poles (7.2642, 18.0967) (7.3776, 18.2172) (7.3776, 18.4035) knots 0 0 0 1 1 1
  spline S289 degree 2 poles (6.8571, 17.9188) (7.1508, 17.9761) (7.2642, 18.0967) knots 0 0 0 1 1 1
  line L97 (6.9861, 16.9471) -> (6.8571, 17.9188)
  spline S290 degree 2 poles (7.5292, 17.2205) (7.3131, 17.0426) (6.9861, 16.9471) knots 0 0 0 1 1 1
  spline S291 degree 2 poles (7.8575, 17.6741) (7.7453, 17.3983) (7.5292, 17.2205) knots 0 0 0 1 1 1
  spline S292 degree 2 poles (7.9697, 18.4273) (7.9697, 17.9498) (7.8575, 17.6741) knots 0 0 0 1 1 1
  spline S293 degree 2 poles (7.8181, 19.2176) (7.9697, 18.9168) (7.9697, 18.4273) knots 0 0 0 1 1 1
  spline S294 degree 2 poles (7.386, 19.6783) (7.6665, 19.5184) (7.8181, 19.2176) knots 0 0 0 1 1 1
  spline S295 degree 2 poles (6.7998, 19.8383) (7.1054, 19.8383) (7.386, 19.6783) knots 0 0 0 1 1 1
  spline S296 degree 2 poles (6.3808, 19.7416) (6.5563, 19.8383) (6.7998, 19.8383) knots 0 0 0 1 1 1
  spline S297 degree 2 poles (6.0979, 19.4706) (6.2054, 19.6449) (6.3808, 19.7416) knots 0 0 0 1 1 1
  spline S298 degree 2 poles (5.9809, 19.1603) (6.0311, 19.3632) (6.0979, 19.4706) knots 0 0 0 1 1 1
  spline S299 degree 2 poles (5.6586, 19.5351) (5.8425, 19.411) (5.9809, 19.1603) knots 0 0 0 1 1 1
  spline S300 degree 2 poles (5.248, 19.6592) (5.4748, 19.6592) (5.6586, 19.5351) knots 0 0 0 1 1 1
  spline S301 degree 2 poles (4.6058, 19.3537) (4.8612, 19.6592) (5.248, 19.6592) knots 0 0 0 1 1 1
  spline S302 degree 2 poles (4.3503, 18.3629) (4.3503, 19.0481) (4.6058, 19.3537) knots 0 0 0 1 1 1
  spline S303 degree 2 poles (4.5843, 17.4401) (4.3503, 17.766) (4.3503, 18.3629) knots 0 0 0 1 1 1
  spline S304 degree 2 poles (5.2575, 16.9996) (4.8183, 17.1142) (4.5843, 17.4401) knots 0 0 0 1 1 1
  line L98 (5.4223, 17.9188) -> (5.2575, 16.9996)
  spline S305 degree 2 poles (5.0582, 18.0644) (5.162, 17.957) (5.4223, 17.9188) knots 0 0 0 1 1 1
  spline S306 degree 2 poles (8.9543, 18.3438) (8.9543, 18.1719) (9.0582, 18.0644) knots 0 0 0 1 1 1
  spline S307 degree 2 poles (9.0498, 18.6064) (8.9543, 18.5109) (8.9543, 18.3438) knots 0 0 0 1 1 1
  spline S308 degree 2 poles (9.3053, 18.7019) (9.1453, 18.7019) (9.0498, 18.6064) knots 0 0 0 1 1 1
  spline S309 degree 2 poles (9.5942, 18.5742) (9.4724, 18.7019) (9.3053, 18.7019) knots 0 0 0 1 1 1
  spline S310 degree 2 poles (9.7159, 18.2554) (9.7159, 18.4464) (9.5942, 18.5742) knots 0 0 0 1 1 1
  spline S311 degree 2 poles (9.704, 18.1289) (9.7159, 18.2101) (9.7159, 18.2554) knots 0 0 0 1 1 1
  line L99 (10.3987, 18.0788) -> (9.704, 18.1289)
  spline S312 degree 2 poles (10.3414, 18.3939) (10.3414, 18.2793) (10.3987, 18.0788) knots 0 0 0 1 1 1
  spline S313 degree 2 poles (10.4751, 18.7341) (10.3414, 18.6088) (10.3414, 18.3939) knots 0 0 0 1 1 1
  spline S314 degree 2 poles (10.8524, 18.8595) (10.6088, 18.8595) (10.4751, 18.7341) knots 0 0 0 1 1 1
  spline S315 degree 2 poles (11.2344, 18.7293) (11.0911, 18.8595) (10.8524, 18.8595) knots 0 0 0 1 1 1
  spline S316 degree 2 poles (11.3776, 18.4035) (11.3776, 18.5992) (11.2344, 18.7293) knots 0 0 0 1 1 1
  spline S317 degree 2 poles (11.2642, 18.0967) (11.3776, 18.2172) (11.3776, 18.4035) knots 0 0 0 1 1 1
  spline S318 degree 2 poles (10.8571, 17.9188) (11.1508, 17.9761) (11.2642, 18.0967) knots 0 0 0 1 1 1
  line L100 (10.9861, 16.9471) -> (10.8571, 17.9188)
  spline S319 degree 2 poles (11.5292, 17.2205) (11.3131, 17.0426) (10.9861, 16.9471) knots 0 0 0 1 1 1
  spline S320 degree 2 poles (11.8575, 17.6741) (11.7453, 17.3983) (11.5292, 17.2205) knots 0 0 0 1 1 1
  spline S321 degree 2 poles (11.9697, 18.4273) (11.9697, 17.9498) (11.8575, 17.6741) knots 0 0 0 1 1 1
  spline S322 degree 2 poles (11.8181, 19.2176) (11.9697, 18.9168) (11.9697, 18.4273) knots 0 0 0 1 1 1
  spline S323 degree 2 poles (11.386, 19.6783) (11.6665, 19.5184) (11.8181, 19.2176) knots 0 0 0 1 1 1
  spline S324 degree 2 poles (10.7998, 19.8383) (11.1054, 19.8383) (11.386, 19.6783) knots 0 0 0 1 1 1
  spline S325 degree 2 poles (10.3808, 19.7416) (10.5563, 19.8383) (10.7998, 19.8383) knots 0 0 0 1 1 1
  spline S326 degree 2 poles (10.0979, 19.4706) (10.2054, 19.6449) (10.3808, 19.7416) knots 0 0 0 1 1 1
  spline S327 degree 2 poles (9.9809, 19.1603) (10.0311, 19.3632) (10.0979, 19.4706) knots 0 0 0 1 1 1
  spline S328 degree 2 poles (9.6586, 19.5351) (9.8425, 19.411) (9.9809, 19.1603) knots 0 0 0 1 1 1
  spline S329 degree 2 poles (9.248, 19.6592) (9.4748, 19.6592) (9.6586, 19.5351) knots 0 0 0 1 1 1
  spline S330 degree 2 poles (8.6058, 19.3537) (8.8612, 19.6592) (9.248, 19.6592) knots 0 0 0 1 1 1
  spline S331 degree 2 poles (8.3503, 18.3629) (8.3503, 19.0481) (8.6058, 19.3537) knots 0 0 0 1 1 1
  spline S332 degree 2 poles (8.5843, 17.4401) (8.3503, 17.766) (8.3503, 18.3629) knots 0 0 0 1 1 1
  spline S333 degree 2 poles (9.2575, 16.9996) (8.8183, 17.1142) (8.5843, 17.4401) knots 0 0 0 1 1 1
  line L101 (9.4223, 17.9188) -> (9.2575, 16.9996)
  spline S334 degree 2 poles (9.0582, 18.0644) (9.162, 17.957) (9.4223, 17.9188) knots 0 0 0 1 1 1
  spline S335 degree 2 poles (-1.2431, 21.3042) (-1.5225, 21.3042) (-1.6729, 21.4415) knots -1 -1 -1 0 0 0
  spline S336 degree 2 poles (-1.6729, 21.4415) (-1.8233, 21.5788) (-1.8233, 21.7817) knots -1 -1 -1 0 0 0
  spline S337 degree 2 poles (-1.8233, 21.7817) (-1.8233, 21.9798) (-1.6681, 22.1135) knots -1 -1 -1 0 0 0
  spline S338 degree 2 poles (-1.6681, 22.1135) (-1.5129, 22.2472) (-1.2169, 22.2472) knots -1 -1 -1 0 0 0
  spline S339 degree 2 poles (-1.2169, 22.2472) (-0.928, 22.2472) (-0.7824, 22.1183) knots -1 -1 -1 0 0 0
  spline S340 degree 2 poles (-0.7824, 22.1183) (-0.6367, 21.9894) (-0.6367, 21.7984) knots -1 -1 -1 0 0 0
  spline S341 degree 2 poles (-0.6367, 21.7984) (-0.6367, 21.5907) (-0.7979, 21.4474) knots -1 -1 -1 0 0 0
  spline S342 degree 2 poles (-0.7979, 21.4474) (-0.959, 21.3042) (-1.2431, 21.3042) knots -1 -1 -1 0 0 0
  spline S343 degree 2 poles (-3.553, 22.449) (-3.4563, 22.6913) (-3.2701, 22.8513) knots 0 0 0 1 1 1
  spline S344 degree 2 poles (-3.6497, 21.7889) (-3.6497, 22.2067) (-3.553, 22.449) knots 0 0 0 1 1 1
  spline S345 degree 2 poles (-3.2092, 20.6835) (-3.6497, 21.0822) (-3.6497, 21.7889) knots 0 0 0 1 1 1
  spline S346 degree 2 poles (-1.8209, 20.2848) (-2.7687, 20.2848) (-3.2092, 20.6835) knots 0 0 0 1 1 1
  spline S347 degree 2 poles (-0.7812, 20.4746) (-1.1739, 20.2848) (-1.8209, 20.2848) knots 0 0 0 1 1 1
  spline S348 degree 2 poles (-0.2094, 20.9819) (-0.3884, 20.6644) (-0.7812, 20.4746) knots 0 0 0 1 1 1
  spline S349 degree 2 poles (-0.0303, 21.8247) (-0.0303, 21.2994) (-0.2094, 20.9819) knots 0 0 0 1 1 1
  spline S350 degree 2 poles (-0.1771, 22.5516) (-0.0303, 22.2616) (-0.0303, 21.8247) knots 0 0 0 1 1 1
  spline S351 degree 2 poles (-0.6105, 23.0053) (-0.324, 22.8417) (-0.1771, 22.5516) knots 0 0 0 1 1 1
  spline S352 degree 2 poles (-1.2431, 23.1688) (-0.897, 23.1688) (-0.6105, 23.0053) knots 0 0 0 1 1 1
  spline S353 degree 2 poles (-2.0907, 22.8453) (-1.7564, 23.1688) (-1.2431, 23.1688) knots 0 0 0 1 1 1
  spline S354 degree 2 poles (-2.4249, 22.0539) (-2.4249, 22.5218) (-2.0907, 22.8453) knots 0 0 0 1 1 1
  spline S355 degree 2 poles (-2.3402, 21.6289) (-2.4249, 21.8127) (-2.4249, 22.0539) knots 0 0 0 1 1 1
  spline S356 degree 2 poles (-2.0787, 21.2708) (-2.2554, 21.4451) (-2.3402, 21.6289) knots 0 0 0 1 1 1
  spline S357 degree 2 poles (-2.8141, 21.4116) (-2.6422, 21.3161) (-2.0787, 21.2708) knots 0 0 0 1 1 1
  spline S358 degree 2 poles (-3.0528, 21.7793) (-3.0528, 21.5429) (-2.8141, 21.4116) knots 0 0 0 1 1 1
  spline S359 degree 2 poles (-2.9693, 22.0001) (-3.0528, 21.9106) (-3.0528, 21.7793) knots 0 0 0 1 1 1
  spline S360 degree 2 poles (-2.6828, 22.1279) (-2.8857, 22.0897) (-2.9693, 22.0001) knots 0 0 0 1 1 1
  line L102 (-2.8021, 23.0948) -> (-2.6828, 22.1279)
  spline S361 degree 2 poles (-3.2701, 22.8513) (-3.0839, 23.0112) (-2.8021, 23.0948) knots 0 0 0 1 1 1
  line L103 (14.5014, 18.7186) -> (14.5014, 17.7826)
  line L104 (14.5014, 17.7826) -> (13.3999, 18.7186)
  line L105 (13.3999, 18.7186) -> (14.5014, 18.7186)
  line L106 (15.91, 19.5661) -> (15.91, 18.7186)
  line L107 (15.2558, 19.5661) -> (15.91, 19.5661)
  line L108 (15.2558, 20.0054) -> (15.2558, 19.5661)
  line L109 (14.5014, 20.0054) -> (15.2558, 20.0054)
  line L110 (14.5014, 19.5661) -> (14.5014, 20.0054)
  line L111 (12.3503, 19.5661) -> (14.5014, 19.5661)
  line L112 (12.3503, 18.7186) -> (12.3503, 19.5661)
  line L113 (14.456, 16.9471) -> (12.3503, 18.7186)
  line L114 (15.2558, 16.9471) -> (14.456, 16.9471)
  line L115 (15.2558, 18.7186) -> (15.2558, 16.9471)
  line L116 (15.91, 18.7186) -> (15.2558, 18.7186)
  spline S362 degree 2 poles (10.8476, 21.2063) (10.6041, 21.2063) (10.4608, 21.3412) knots -1 -1 -1 0 0 0
  spline S363 degree 2 poles (10.4608, 21.3412) (10.3176, 21.4761) (10.3176, 21.6575) knots -1 -1 -1 0 0 0
  spline S364 degree 2 poles (10.3176, 21.6575) (10.3176, 21.8414) (10.4656, 21.981) knots -1 -1 -1 0 0 0
  spline S365 degree 2 poles (10.4656, 21.981) (10.6136, 22.1207) (10.8452, 22.1207) knots -1 -1 -1 0 0 0
  spline S366 degree 2 poles (10.8452, 22.1207) (11.0744, 22.1207) (11.2236, 21.9822) knots -1 -1 -1 0 0 0
  spline S367 degree 2 poles (11.2236, 21.9822) (11.3728, 21.8438) (11.3728, 21.6695) knots -1 -1 -1 0 0 0
  spline S368 degree 2 poles (11.3728, 21.6695) (11.3728, 21.488) (11.226, 21.3472) knots -1 -1 -1 0 0 0
  spline S369 degree 2 poles (11.226, 21.3472) (11.0792, 21.2063) (10.8476, 21.2063) knots -1 -1 -1 0 0 0
  spline S370 degree 2 poles (9.3411, 21.2588) (9.1644, 21.2588) (9.0534, 21.3699) knots -1 -1 -1 0 0 0
  spline S371 degree 2 poles (9.0534, 21.3699) (8.9424, 21.4809) (8.9424, 21.6575) knots -1 -1 -1 0 0 0
  spline S372 degree 2 poles (8.9424, 21.6575) (8.9424, 21.8318) (9.0558, 21.944) knots -1 -1 -1 0 0 0
  spline S373 degree 2 poles (9.0558, 21.944) (9.1692, 22.0562) (9.3507, 22.0562) knots -1 -1 -1 0 0 0
  spline S374 degree 2 poles (9.3507, 22.0562) (9.5249, 22.0562) (9.6348, 21.9488) knots -1 -1 -1 0 0 0
  spline S375 degree 2 poles (9.6348, 21.9488) (9.7446, 21.8414) (9.7446, 21.6743) knots -1 -1 -1 0 0 0
  spline S376 degree 2 poles (9.7446, 21.6743) (9.7446, 21.4856) (9.6336, 21.3722) knots -1 -1 -1 0 0 0
  spline S377 degree 2 poles (9.6336, 21.3722) (9.5226, 21.2588) (9.3411, 21.2588) knots -1 -1 -1 0 0 0
  spline S378 degree 2 poles (10.881, 20.237) (10.573, 20.237) (10.3594, 20.3803) knots 0 0 0 1 1 1
  spline S379 degree 2 poles (11.4516, 20.3898) (11.1962, 20.237) (10.881, 20.237) knots 0 0 0 1 1 1
  spline S380 degree 2 poles (11.8384, 20.8363) (11.7071, 20.5426) (11.4516, 20.3898) knots 0 0 0 1 1 1
  spline S381 degree 2 poles (11.9697, 21.6862) (11.9697, 21.1299) (11.8384, 20.8363) knots 0 0 0 1 1 1
  spline S382 degree 2 poles (11.9112, 22.2437) (11.9697, 21.9822) (11.9697, 21.6862) knots 0 0 0 1 1 1
  spline S383 degree 2 poles (11.7286, 22.6806) (11.8527, 22.5051) (11.9112, 22.2437) knots 0 0 0 1 1 1
  spline S384 degree 2 poles (11.3764, 22.9766) (11.6044, 22.856) (11.7286, 22.6806) knots 0 0 0 1 1 1
  spline S385 degree 2 poles (10.8858, 23.0972) (11.1484, 23.0972) (11.3764, 22.9766) knots 0 0 0 1 1 1
  spline S386 degree 2 poles (10.3892, 22.9575) (10.6136, 23.0972) (10.8858, 23.0972) knots 0 0 0 1 1 1
  spline S387 degree 2 poles (10.0287, 22.5337) (10.1648, 22.8178) (10.3892, 22.9575) knots 0 0 0 1 1 1
  spline S388 degree 2 poles (9.7326, 22.8489) (9.8854, 22.7486) (10.0287, 22.5337) knots 0 0 0 1 1 1
  spline S389 degree 2 poles (9.291, 22.9826) (9.5273, 22.9826) (9.7326, 22.8489) knots 0 0 0 1 1 1
  spline S390 degree 2 poles (8.6177, 22.6471) (8.8851, 22.9826) (9.291, 22.9826) knots 0 0 0 1 1 1
  spline S391 degree 2 poles (8.3503, 21.6098) (8.3503, 22.3117) (8.6177, 22.6471) knots 0 0 0 1 1 1
  spline S392 degree 2 poles (8.5652, 20.7575) (8.3503, 21.0798) (8.3503, 21.6098) knots 0 0 0 1 1 1
  spline S393 degree 2 poles (9.2838, 20.3444) (8.8445, 20.3444) (8.5652, 20.7575) knots 0 0 0 1 1 1
  spline S394 degree 2 poles (9.7565, 20.4877) (9.5512, 20.3444) (9.2838, 20.3444) knots 0 0 0 1 1 1
  spline S395 degree 2 poles (10.0287, 20.8219) (9.9069, 20.5927) (9.7565, 20.4877) knots 0 0 0 1 1 1
  spline S396 degree 2 poles (10.3594, 20.3803) (10.1457, 20.5235) (10.0287, 20.8219) knots 0 0 0 1 1 1
  line L117 (15.1174, 21.6361) -> (15.1174, 23.1545)
  spline S397 degree 2 poles (14.9049, 21.8688) (14.9861, 21.7698) (15.1174, 21.6361) knots 0 0 0 1 1 1
  spline S398 degree 2 poles (14.6208, 22.2616) (14.8237, 21.9679) (14.9049, 21.8688) knots 0 0 0 1 1 1
  spline S399 degree 2 poles (13.9809, 22.9432) (14.2722, 22.7558) (14.6208, 22.2616) knots 0 0 0 1 1 1
  spline S400 degree 2 poles (13.3698, 23.1306) (13.6897, 23.1306) (13.9809, 22.9432) knots 0 0 0 1 1 1
  spline S401 degree 2 poles (12.8266, 22.9671) (13.0689, 23.1306) (13.3698, 23.1306) knots 0 0 0 1 1 1
  spline S402 degree 2 poles (12.4673, 22.5182) (12.5843, 22.8035) (12.8266, 22.9671) knots 0 0 0 1 1 1
  spline S403 degree 2 poles (12.3503, 21.7196) (12.3503, 22.2329) (12.4673, 22.5182) knots 0 0 0 1 1 1
  spline S404 degree 2 poles (12.4733, 20.9497) (12.3503, 21.2278) (12.3503, 21.7196) knots 0 0 0 1 1 1
  spline S405 degree 2 poles (12.8266, 20.5187) (12.5962, 20.6715) (12.4733, 20.9497) knots 0 0 0 1 1 1
  spline S406 degree 2 poles (13.4676, 20.3086) (13.057, 20.3659) (12.8266, 20.5187) knots 0 0 0 1 1 1
  line L118 (13.5464, 21.2827) -> (13.4676, 20.3086)
  spline S407 degree 2 poles (13.1334, 21.4415) (13.2504, 21.3233) (13.5464, 21.2827) knots 0 0 0 1 1 1
  spline S408 degree 2 poles (13.0164, 21.7459) (13.0164, 21.5597) (13.1334, 21.4415) knots 0 0 0 1 1 1
  spline S409 degree 2 poles (13.1298, 22.0431) (13.0164, 21.9249) (13.0164, 21.7459) knots 0 0 0 1 1 1
  spline S410 degree 2 poles (13.4032, 22.1613) (13.2432, 22.1613) (13.1298, 22.0431) knots 0 0 0 1 1 1
  spline S411 degree 2 poles (13.7159, 22.0419) (13.5512, 22.1613) (13.4032, 22.1613) knots 0 0 0 1 1 1
  spline S412 degree 2 poles (14.1982, 21.4952) (13.8807, 21.9225) (13.7159, 22.0419) knots 0 0 0 1 1 1
  spline S413 degree 2 poles (15.0971, 20.5414) (14.7163, 20.7957) (14.1982, 21.4952) knots 0 0 0 1 1 1
  spline S414 degree 2 poles (15.91, 20.237) (15.4779, 20.2871) (15.0971, 20.5414) knots 0 0 0 1 1 1
  line L119 (15.91, 23.1545) -> (15.91, 20.237)
  line L120 (15.1174, 23.1545) -> (15.91, 23.1545)
  spline S415 degree 2 poles (0.9543, 18.3438) (0.9543, 18.1719) (1.0582, 18.0644) knots 0 0 0 1 1 1